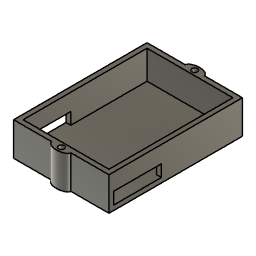
ADC (Autodesk Fusion 360 design; units mm, degrees)
Autodesk Fusion 360 part; units mm, degrees
note: some values were not read from the file. Set by a fixed rule: which sketch regions a step uses.
sketch "Boceto1" plane through (0, 0, 0) normal (0, 0, 1) x (1, 0, 0)
  line L0 (10, -14) -> (-10, -14)
  line L1 (-10, -14) -> (-10, 14)
  line L2 (-10, 14) -> (10, 14)
  line L3 (10, 14) -> (10, -14)
  line L4 (10, -14) -> (-10, 14) construction
  line L5 (-10, -14) -> (10, 14) construction
  line L6 (9, -13) -> (-9, -13)
  line L7 (-9, -13) -> (-9, 13)
  line L8 (-9, 13) -> (9, 13)
  line L9 (9, 13) -> (9, -13)
  line L10 (9, -13) -> (-9, 13) construction
  line L11 (-9, -13) -> (9, 13) construction
  dimension "d1" = 20
  dimension "d2" = 28
  dimension "d3" = 18
  dimension "d4" = 26
  constraint horizontal L0
  constraint perpendicular L0 L1
  constraint parallel L0 L2
  constraint parallel L1 L3
  constraint coincident L4 origin
  constraint coincident L5 origin
  constraint horizontal L6
  constraint perpendicular L6 L7
  constraint parallel L6 L8
  constraint parallel L7 L9
  constraint coincident L10 origin
  constraint coincident L11 origin
  measures "d1" distance of L1.end L2.end
  measures "d2" distance of L0.end L1.end
  measures "d3" distance of L7.end L8.end
  measures "d4" distance of L6.end L7.end
extrude "Extruir1" add sketch "Boceto1" against normal blind 1 contours L0 L1 L2 L3 | L6 L7 L8 L9
extrude "Extruir2" add sketch "Boceto1" along normal blind 6
sketch "Boceto2" plane through (10, 0, 0) normal (1, 0, 0) x (0, 1, 0)
  line L0 (-14, 6) -> (-14, -1)
  line L1 (-14, -1) -> (14, -1)
  line L2 (14, -1) -> (14, 6)
  line L3 (14, 6) -> (-14, 6)
  line L4 (13, 6) -> (-13, 6)
  line L5 (-13, 6) -> (13, 6)
  line L6 (14, 6) -> (-14, 6)
  line L7 (-14, 6) -> (14, 6)
  line L8 (-13, 0) -> (13, 0)
  line L9 (13, 0) -> (13, 6)
  line L10 (13, 6) -> (-13, 6)
  line L11 (-13, 6) -> (-13, 0)
  line L12 (-13, 0) -> (-3, 0)
  line L13 (-3, 0) -> (-2.997, 6)
  line L14 (-13, 6) -> (-2.997, 6)
  line L15 (-13, 0) -> (-13, 2.5)
  line L16 (-13, 2.5) -> (-2.9987, 2.4949)
  line L17 (-2.9987, 2.4949) -> (-3, 0)
  dimension "d9" = 10
  dimension "d12" = 2.5
  constraint coincident L8.start L11.end
  constraint perpendicular L0 L12
  constraint coincident L5 L13.end
  constraint coincident L4.end L5.start
  constraint parallel L5 L14
  constraint perpendicular L8 L15
  constraint coincident L13 L16.end
  constraint perpendicular L13 L16
  measures "d9" distance of L8.start L12.end
  measures "d12" distance of L8.start L15.end
extrude "Extruir3" cut sketch "Boceto2" against normal blind 28 contours L8 L11 L12 L13 L15 L16 L17
sketch "Boceto3" plane through (0, 0, 6) normal (0, 0, 1) x (-1, 0, 0)
  line L0 (9, -13) -> (-9, -13)
  line L1 (-9, -13) -> (-9, 13)
  line L2 (-9, 13) -> (9, 13)
  line L3 (9, 13) -> (9, -13)
  line L4 (-10, -14) -> (10, -14)
  line L5 (10, -14) -> (10, 14)
  line L6 (10, 14) -> (-10, 14)
  line L7 (-10, 14) -> (-10, -14)
  line L8 (0, -14) -> (2, -14) construction
  ellipse E0 centre (0, -14) end of major axis (2, -14) minor radius 1
  line L9 (0, -15) -> (0, -13) construction
  line L10 (0, 14) -> (2, 14) construction
  ellipse E1 centre (0, 14) end of major axis (2, 14) minor radius 1
  line L11 (-2, 14) -> (2, 14) construction
  line L12 (0, 13) -> (0, 15) construction
  circle A0 centre (0, 14) radius 0.6
  circle A1 centre (0, -14) radius 0.6
  dimension "d15" = 2
  dimension "d17" = 2
  dimension "d18" = 2
  dimension "d19" = 2
  dimension "d20" = 1.2
  dimension "d21" = 1.2
  constraint midpoint L4 L8.start
  constraint coincident E0 L9.start
  constraint coincident E0 L9.end
  constraint coincident L8.start E0.centre
  constraint midpoint L6 L10.start
  constraint parallel L6 L10
  constraint coincident E1 L11.start
  constraint coincident E1 L10.end
  constraint coincident E1 L12.start
  constraint coincident E1 L12.end
  constraint coincident L10.start E1.centre
  constraint coincident L10.end L11.end
  constraint concentric E0 A1
  measures "d15" distance of L8.start L8.end
  measures "d17" distance of E0
  measures "d18" distance of L10.start L10.end
  measures "d19" distance of E1
  measures "d20" diameter of A0
  measures "d21" diameter of A1
extrude "Extruir4" add sketch "Boceto3" against normal blind 7 contours L4 E0 A1 | L4 A1 | L6 E1 A0 | L6 A0 picked at (-1.4687, -14.1432) picked at (-0.0731, -14.1862) picked at (1.4687, 14.1432) picked at (0.1247, 14.1564)
extrude "Extruir5" cut sketch "Boceto3" against normal blind 5 contours L4 A1 | L4 A1 | L6 A0 | L6 A0
